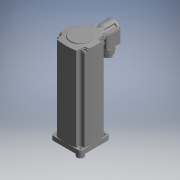
# Autodesk Inventor part: 4808568 EMMT-AS-60-LB---(high_h)
Saved by Autodesk Inventor 2017.3 (Build 213256000, 256)
## iProperties
Part Number: 4808568 EMMT-AS-60-LB---(high_h)
Material: Generic
Catalog Web Link: www.cadenas.de
Description: EMMT-AS (H)-servo motor
Vendor: FESTO
Document SubType Name: Modeling
Designer: partserver
Manufacturer: FESTO
Mass: 654.326 g
Surface Area: 634.047 cm^2
Volume: 654.326 cm^3
Density: 1 g/cm^3
Appearance: PSOLRGB-175-175-175
Category: PARTsolutions
Company: FESTO
Title: 4808568 EMMT-AS-60-LB---(high_h)
Author: Cadenas PARTsolutions
Comments: servo motor
PSOL_IDENT_0: {$CADENAS_DATA\23d-libs\festo\parts\e\emmt\parts\emmt_as.prj},229 {VTYP=3D},{NB=4808568 EMMT-AS-60-L
PSOL_IDENT_1: B---(high_h)},{LINA=4808568 EMMT-AS-60-LB---(high_h)},{NN=EMMT-AS (H)},{DATE=10.08.2021 16:37:16},{G
PSOL_IDENT_2: EOMDATE=08.06.2021 12:24:00},{VERSION=},{LINEID=10},{WBVAR=BAU,WEL,BRE,LODLEVEL},{WBNUMERIC=}  {NB=4
PSOL_IDENT_3: 808568 EMMT-AS-60-LB---(high_h)},{LINA=4808568 EMMT-AS-60-LB---(high_h)},{KT=DUMMY},{TNR=4808568},{T
PSOL_IDENT_4: YP=EMMT-AS},{FLA=60},{BAU=L},{WEL=-},{BRE=B},{LODDEST=mechanical},{LODLEVEL=high},{LODLEVELX='high',
PSOL_IDENT_5: 'High', 'medium', 'Medium','low','Low'},{B1=62},{B2=28},{D1=14},{D2=15},{D3=50},{D4=5},{D5=4.300},{
PSOL_IDENT_6: D6=70},{H1=102},{H3=57},{L=217.300},{L1=187.300},{L2=30},{L3=2.500},{L4=9},{L5=18.400},{L6=44.700},{
PSOL_IDENT_7: L7=14.000},{T1=12.500},{R1=6.000},{WELNB=},{BRENB=B},{BAU1='S','M','L'},{A1=59.000},{R2=90.000},{R3=
PSOL_IDENT_8: 4.000},{R4=0.750},{A2=3.500},{A3=41.274},{R5=1.000},{R6=22.100},{R7=16.900},{R8=15.000},{A4=6.400},{
PSOL_IDENT_9: A5=28.500},{A6=26.500},{A7=4.000},{R9=4.400},{A8=2.400},{R10=2.650},{A9=17.000},{A10=5.500},{R11=2.5
PSOL_IDENT_10: 00},{A11=17.000},{A12=9.000},{Y1=35.000},{X1=52.400},{R12=3.300},{T2=3.400},{T3=1.000},{R13=2.750},{
PSOL_IDENT_11: T4=8.800},{Y2=6.400},{H4=2.400},{H5=31.500},{Y3=31.900},{Y4=8.500},{Y5=13.880},{A13=1.500},{A14=0.35
PSOL_IDENT_12: 0},{A15=1.000},{SC1=1.600}
NB: 4808568 EMMT-AS-60-LB---(high_h)
NN: EMMT-AS (H)
NT: servo motor
NBSYN: $TNR. $TYP.-$FLA.-$BAU.$WELNB.$BRENB.---($LODLEVEL._h)
LINA: 4808568 EMMT-AS-60-LB---(high_h)
CATALOG: Festo
TNR: 4808568
TYP: EMMT-AS
FLA: 60
BAU: L
WEL: -
BRE: B
LODLEVEL: High
B1: 62
B2: 28
D1: 14
D2: 15
D3: 50
D4: 5
D5: 4.3
D6: 70
H1: 102
H3: 57
L2: 30
L3: 2.5
L4: 9
L5: 18.4
L6: 44.7
L7: 14
T1: 12.5
R1: 6
A1: 59
R2: 90
R3: 4
R4: 0.75
A2: 3.5
A3: 41.274
R5: 1
R6: 22.1
R7: 16.9
R8: 15
A4: 6.4
A5: 28.5
A6: 26.5
A7: 4
R9: 4.4
A8: 2.4
R10: 2.65
A9: 17
A10: 5.5
R11: 2.5
A11: 17
A12: 9
Y1: 35
X1: 52.4
R12: 3.3
T2: 3.4
T3: 1
R13: 2.75
T4: 8.8
Y2: 6.4
H4: 2.4
H5: 31.5
Y3: 31.9
Y4: 8.5
Y5: 13.88
A13: 1.5
A14: 0.35
A15: 1
SC1: 1.6
SUPPLIER: FESTO
ARTICLENO: 4808568 EMMT-AS-60-LB---(high_h)
BOMINFO: 4808568 EMMT-AS-60-LB---(high_h)
CREATOR: CADENAS GmbH
Autodesk Inventor part; units mm, degrees
sketch "Sketch_1" plane through (0, 0, 0) normal (0, 0, 1) x (1, 0, 0)
  line L0 (-31, 25) -> (-31, -25)
  arc A0 (-31, -25) -> (-25, -31) centre (-25, -25) ccw
  line L1 (-25, -31) -> (25, -31)
  arc A1 (25, -31) -> (31, -25) centre (25, -25) ccw
  line L2 (31, -25) -> (31, 25)
  arc A2 (31, 25) -> (25, 31) centre (25, 25) ccw
  line L3 (25, 31) -> (-25, 31)
  arc A3 (-25, 31) -> (-31, 25) centre (-25, 25) ccw
  constraints: 8 end point, 8 point on circle, 4 centre point
extrude "Extrusion1" add sketch "Sketch_1" against normal blind 9
sketch "Sketch_2" plane through (0, 0, 0) normal (0.7071068, -0.7071068, 0) x (0, 0, -1)
  line L0 (9, 35) -> (0, 35)
  line L1 (0, 35) -> (0, 37.65)
  line L2 (0, 37.65) -> (0.5, 37.15)
  line L3 (0.5, 37.15) -> (8.5, 37.15)
  line L4 (8.5, 37.15) -> (9, 37.65)
  line L5 (9, 37.65) -> (9, 35)
  line L6 (9, 35) -> (0, 35)
  constraints: 14 end point
revolve "Revolution1" cut sketch "Sketch_2" angle 360 about axis through (24.7487, 24.7487, -9) along (0, 0, -1)
pattern_linear "Rectangular Pattern1" count 2 spacing 49.4975 along (-1, 0, 0) count 2 spacing 49.4975 along (0, -1, 0) of "Revolution1"
sketch "Sketch_4" plane through (0, 0, -9) normal (0, 0, 1) x (1, 0, 0)
  arc A0 (-28.8206, 19.686) -> (-28.8206, -19.686) centre (59, 0) ccw
  arc A1 (-28.8206, -19.686) -> (-28.1932, -20.2647) centre (-28.0888, -19.522) ccw
  line L0 (-28.1932, -20.2647) -> (-23.6462, -20.9037)
  arc A2 (-20.9037, -23.6462) -> (-23.6462, -20.9037) centre (-24.7487, -24.7487) ccw
  line L1 (-20.9037, -23.6462) -> (-20.2647, -28.1932)
  arc A3 (-20.2647, -28.1932) -> (-19.686, -28.8206) centre (-19.522, -28.0888) ccw
  arc A4 (-19.686, -28.8206) -> (19.686, -28.8206) centre (0, 59) ccw
  arc A5 (19.686, -28.8206) -> (20.2647, -28.1932) centre (19.522, -28.0888) ccw
  line L2 (20.2647, -28.1932) -> (20.9037, -23.6462)
  arc A6 (23.6462, -20.9037) -> (20.9037, -23.6462) centre (24.7487, -24.7487) ccw
  line L3 (23.6462, -20.9037) -> (28.1932, -20.2647)
  arc A7 (28.1932, -20.2647) -> (28.8206, -19.686) centre (28.0888, -19.522) ccw
  arc A8 (28.8206, -19.686) -> (28.8206, 19.686) centre (-59, 0) ccw
  arc A9 (28.8206, 19.686) -> (28.1932, 20.2647) centre (28.0888, 19.522) ccw
  line L4 (28.1932, 20.2647) -> (23.6462, 20.9037)
  arc A10 (20.9037, 23.6462) -> (23.6462, 20.9037) centre (24.7487, 24.7487) ccw
  line L5 (20.9037, 23.6462) -> (20.2647, 28.1932)
  arc A11 (20.2647, 28.1932) -> (19.686, 28.8206) centre (19.522, 28.0888) ccw
  arc A12 (19.686, 28.8206) -> (-19.686, 28.8206) centre (0, -59) ccw
  arc A13 (-19.686, 28.8206) -> (-20.2647, 28.1932) centre (-19.522, 28.0888) ccw
  line L6 (-20.2647, 28.1932) -> (-20.9037, 23.6462)
  arc A14 (-23.6462, 20.9037) -> (-20.9037, 23.6462) centre (-24.7487, 24.7487) ccw
  line L7 (-23.6462, 20.9037) -> (-28.1932, 20.2647)
  arc A15 (-28.1932, 20.2647) -> (-28.8206, 19.686) centre (-28.0888, 19.522) ccw
  constraints: 32 point on circle, 16 centre point, 16 end point
extrude "Extrusion2" add sketch "Sketch_4" against normal blind 178.3
sketch "Sketch_5" plane through (0, 0, 0) normal (1, 0, 0) x (0, 1, 0)
  line L0 (0, -187.3) -> (0, -183.8)
  line L1 (42.2, -183.8) -> (37.2, -183.8)
  line L2 (37.2, -183.8) -> (21.5433, -185.2731)
  arc A0 (21.5433, -185.2731) -> (20.637, -186.2687) centre (21.637, -186.2687) ccw
  line L3 (20.637, -186.2687) -> (20.637, -186.8)
  arc A1 (20.137, -187.3) -> (20.637, -186.8) centre (20.137, -186.8) ccw
  line L4 (20.137, -187.3) -> (42.2, -187.3)
  line L5 (42.2, -187.3) -> (42.2, -183.8)
  constraints: 12 end point, 4 point on circle, 2 centre point
revolve "Revolution2" cut sketch "Sketch_5" angle 360 about axis through (0, 0, -187.3) along (0, 0, -1)
sketch "Sketch_9" plane through (0, 0, 0) normal (1, 0, 0) x (0, 1, 0)
  line L0 (0, 0) -> (0, 2.5)
  arc A0 (22.35, 2.5) -> (22.1, 2.25) centre (22.35, 2.25) ccw
  line L1 (22.1, 2.25) -> (22.1, 1)
  line L2 (22.1, 1) -> (16.9, 1)
  line L3 (16.9, 1) -> (16.9, 2.25)
  arc A1 (16.9, 2.25) -> (16.65, 2.5) centre (16.65, 2.25) ccw
  line L4 (16.65, 2.5) -> (15.7, 2.5)
  line L5 (15.7, 2.5) -> (15, 1)
  line L6 (15, 1) -> (15, 0)
  line L7 (15, 0) -> (25, 0)
  line L8 (25, 0) -> (25, 2)
  line L9 (25, 2) -> (24.7, 2.5)
  line L10 (24.7, 2.5) -> (22.35, 2.5)
  constraints: 22 end point, 4 point on circle, 2 centre point
revolve "Revolution3" add sketch "Sketch_9" angle 360 about axis through (0, 0, 0) along (0, 0, -1)
sketch "Sketch_22" plane through (0, 0, 0) normal (1, 0, 0) x (0, 1, 0)
  line L0 (0, -6.4) -> (0, 2.5)
  line L1 (0, 2.5) -> (15, 2.5)
  line L2 (15, 2.5) -> (15, -4.9)
  line L3 (15, -4.9) -> (13.25, -4.9)
  arc A0 (13.25, -4.9) -> (13, -5.15) centre (13.25, -5.15) ccw
  line L4 (13, -5.15) -> (13, -6.4)
  line L5 (13, -6.4) -> (0, -6.4)
  line L6 (0, -6.4) -> (0, 2.5)
  constraints: 14 end point, 2 point on circle, 1 centre point
revolve "Revolution4" cut sketch "Sketch_22" angle 360 about axis through (0, 0, -6.4) along (0, 0, -1)
sketch "Sketch_7" plane through (0, 0, 0) normal (1, 0, 0) x (0, 1, 0)
  line L0 (0, -6.4) -> (0, 11.8066)
  line L1 (0, 11.8066) -> (2.067, 13)
  line L2 (2.067, 13) -> (2.067, 25.567)
  line L3 (2.067, 25.567) -> (2.5, 26)
  line L4 (2.5, 26) -> (2.65, 26)
  line L5 (2.65, 26) -> (2.65, 27.6)
  line L6 (2.65, 27.6) -> (4.05, 29.7979)
  line L7 (4.05, 29.7979) -> (4.4, 30)
  line L8 (4.4, 30) -> (6.6, 30)
  line L9 (6.6, 30) -> (7, 29.6)
  line L10 (7, 29.6) -> (7, 3.5)
  line L11 (7, 3.5) -> (6.8136, 2.8045)
  arc A0 (6.8136, 2.8045) -> (6.8, 2.7009) centre (7.2, 2.7009) ccw
  line L12 (6.8, 2.7009) -> (6.8, 1.9)
  arc A1 (6.8, 1.9) -> (7.2, 1.5) centre (7.2, 1.9) ccw
  line L13 (7.2, 1.5) -> (7.3, 1.5)
  arc A2 (7.5, 1.3) -> (7.3, 1.5) centre (7.3, 1.3) ccw
  line L14 (7.5, 1.3) -> (7.5, -6.4)
  line L15 (7.5, -6.4) -> (0, -6.4)
  line L16 (0, -6.4) -> (0, 11.8066)
  constraints: 34 end point, 6 point on circle, 3 centre point
revolve "Revolution5" add sketch "Sketch_7" angle 360 about axis through (0, 0, -6.4) along (0, 0, -1)
thread "Thread1" size "M5x0.8" class "6H" standard "ISO Metric profile" length 12.5 offset 0.5
sketch "Sketch_10" plane through (0, 0, 0) normal (0, 0, 1) x (1, 0, 0)
  arc A0 (-11.05, 19.1392) -> (-8.45, 14.6358) centre (-9.75, 16.8875) ccw
  arc A1 (8.45, 14.6358) -> (-8.45, 14.6358) centre (0, 0) ccw
  arc A2 (8.45, 14.6358) -> (11.05, 19.1392) centre (9.75, 16.8875) ccw
  arc A3 (11.05, 19.1392) -> (-11.05, 19.1392) centre (0, 0) ccw
  constraints: 8 point on circle, 4 centre point
extrude "Extrusion3" cut sketch "Sketch_10" along normal mid plane 8.8
sketch "Sketch_11" plane through (0, 0, 0) normal (0, 0, 1) x (1, 0, 0)
  arc A0 (-19.1392, 11.05) -> (-19.1392, -11.05) centre (0, 0) ccw
  arc A1 (-19.1392, -11.05) -> (-14.6358, -8.45) centre (-16.8875, -9.75) ccw
  arc A2 (-14.6358, 8.45) -> (-14.6358, -8.45) centre (0, 0) ccw
  arc A3 (-14.6358, 8.45) -> (-19.1392, 11.05) centre (-16.8875, 9.75) ccw
  constraints: 8 point on circle, 4 centre point
extrude "Extrusion4" cut sketch "Sketch_11" along normal mid plane 8.8
sketch "Sketch_12" plane through (0, 0, 0) normal (0, 0, 1) x (1, 0, 0)
  arc A0 (-8.45, -14.6358) -> (-11.05, -19.1392) centre (-9.75, -16.8875) ccw
  arc A1 (-11.05, -19.1392) -> (11.05, -19.1392) centre (0, 0) ccw
  arc A2 (11.05, -19.1392) -> (8.45, -14.6358) centre (9.75, -16.8875) ccw
  arc A3 (-8.45, -14.6358) -> (8.45, -14.6358) centre (0, 0) ccw
  constraints: 8 point on circle, 4 centre point
extrude "Extrusion5" cut sketch "Sketch_12" along normal mid plane 8.8
sketch "Sketch_13" plane through (0, 0, 0) normal (0, 0, 1) x (1, 0, 0)
  arc A0 (14.6358, -8.45) -> (19.1392, -11.05) centre (16.8875, -9.75) ccw
  arc A1 (19.1392, -11.05) -> (19.1392, 11.05) centre (0, 0) ccw
  arc A2 (19.1392, 11.05) -> (14.6358, 8.45) centre (16.8875, 9.75) ccw
  arc A3 (14.6358, -8.45) -> (14.6358, 8.45) centre (0, 0) ccw
  constraints: 8 point on circle, 4 centre point
extrude "Extrusion6" cut sketch "Sketch_13" along normal mid plane 8.8
sketch "Sketch_14" plane through (0, 17.5, 0) normal (0, 1, 0) x (1, 0, 0)
  line L0 (26.2, 0) -> (26.2, 1)
  line L1 (26.2, 1) -> (28.4651, 1)
  arc A0 (28.4651, 1) -> (28.764, 1.2739) centre (28.4651, 1.3) ccw
  line L2 (28.764, 1.2739) -> (28.95, 3.4)
  line L3 (28.95, 3.4) -> (29.5, 3.4)
  line L4 (29.5, 3.4) -> (29.5, 0.5)
  line L5 (29.5, 0.5) -> (30, 0)
  line L6 (30, 0) -> (26.2, 0)
  line L7 (26.2, 0) -> (26.2, 1)
  constraints: 16 end point, 2 point on circle, 1 centre point
revolve "Revolution6" cut sketch "Sketch_14" angle 360 about axis through (26.2, 17.5, 0) along (0, 0, 1)
pattern_linear "Rectangular Pattern2" count 2 spacing 52.4 along (-1, 0, 0) count 2 spacing 35 along (0, -1, 0) of "Revolution6"
sketch "Sketch_16" plane through (0, 0, 0) normal (0, 0, 1) x (1, 0, 0)
  arc A0 (25.0379, 17.1436) -> (25.3103, 16.6718) centre (25.2301, 16.94) ccw
  arc A1 (25.9276, 16.3154) -> (25.3103, 16.6718) centre (25.4508, 16.2023) ccw
  arc A2 (25.9276, 16.3154) -> (26.4724, 16.3154) centre (26.2, 16.38) ccw
  arc A3 (27.0897, 16.6718) -> (26.4724, 16.3154) centre (26.9492, 16.2023) ccw
  arc A4 (27.0897, 16.6718) -> (27.3621, 17.1436) centre (27.1699, 16.94) ccw
  arc A5 (27.3621, 17.8564) -> (27.3621, 17.1436) centre (27.6984, 17.5) ccw
  arc A6 (27.3621, 17.8564) -> (27.0897, 18.3282) centre (27.1699, 18.06) ccw
  arc A7 (26.4724, 18.6846) -> (27.0897, 18.3282) centre (26.9492, 18.7977) ccw
  arc A8 (26.4724, 18.6846) -> (25.9276, 18.6846) centre (26.2, 18.62) ccw
  arc A9 (25.3103, 18.3282) -> (25.9276, 18.6846) centre (25.4508, 18.7977) ccw
  arc A10 (25.3103, 18.3282) -> (25.0379, 17.8564) centre (25.2301, 18.06) ccw
  arc A11 (25.0379, 17.1436) -> (25.0379, 17.8564) centre (24.7016, 17.5) ccw
  constraints: 24 point on circle, 12 centre point
extrude "Extrusion7" cut sketch "Sketch_16" against normal blind 2.25
pattern_linear "Rectangular Pattern3" count 2 spacing 52.4 along (-1, 0, 0) count 2 spacing 35 along (0, -1, 0) of "Extrusion7"
sketch "Sketch_18" plane through (0, 0, -187.3) normal (0, 0, 1) x (1, 0, 0)
  line L0 (-36, -36) -> (36, -36)
  line L1 (36, -36) -> (36, 36)
  line L2 (36, 36) -> (-36, 36)
  line L3 (-36, 36) -> (-36, -36)
  arc A0 (-32.2659, 11.5991) -> (-32.2659, -11.5991) centre (59, 0) ccw
  arc A1 (-32.2659, -11.5991) -> (-31.6262, -12.2472) centre (-31.5219, -11.5045) ccw
  line L4 (-31.6262, -12.2472) -> (-25.0296, -13.1743)
  arc A2 (-21.9443, -16.2596) -> (-25.0296, -13.1743) centre (-26.27, -17.5) ccw
  line L5 (-21.9443, -16.2596) -> (-19.9703, -30.3056)
  arc A3 (-19.9703, -30.3056) -> (-19.3856, -30.9344) centre (-19.2276, -30.2012) ccw
  arc A4 (-19.3856, -30.9344) -> (19.3856, -30.9344) centre (0, 59) ccw
  arc A5 (19.3856, -30.9344) -> (19.9703, -30.3056) centre (19.2276, -30.2012) ccw
  line L6 (19.9703, -30.3056) -> (21.9443, -16.2596)
  arc A6 (25.0296, -13.1743) -> (21.9443, -16.2596) centre (26.27, -17.5) ccw
  line L7 (25.0296, -13.1743) -> (31.6262, -12.2472)
  arc A7 (31.6262, -12.2472) -> (32.2659, -11.5991) centre (31.5219, -11.5045) ccw
  arc A8 (32.2659, -11.5991) -> (32.2659, 11.5991) centre (-59, 0) ccw
  arc A9 (32.2659, 11.5991) -> (31.6262, 12.2472) centre (31.5219, 11.5045) ccw
  line L8 (31.6262, 12.2472) -> (25.0296, 13.1743)
  arc A10 (21.9443, 16.2596) -> (25.0296, 13.1743) centre (26.27, 17.5) ccw
  line L9 (21.9443, 16.2596) -> (19.9703, 30.3056)
  arc A11 (19.9703, 30.3056) -> (19.3856, 30.9344) centre (19.2276, 30.2012) ccw
  arc A12 (19.3856, 30.9344) -> (-19.3856, 30.9344) centre (0, -59) ccw
  arc A13 (-19.3856, 30.9344) -> (-19.9703, 30.3056) centre (-19.2276, 30.2012) ccw
  line L10 (-19.9703, 30.3056) -> (-21.9443, 16.2596)
  arc A14 (-25.0296, 13.1743) -> (-21.9443, 16.2596) centre (-26.27, 17.5) ccw
  line L11 (-25.0296, 13.1743) -> (-31.6262, 12.2472)
  arc A15 (-31.6262, 12.2472) -> (-32.2659, 11.5991) centre (-31.5219, 11.5045) ccw
  constraints: 32 point on circle, 24 end point, 16 centre point
extrude "Extrusion8" cut sketch "Sketch_18" along normal blind 4.5
sketch "Sketch_61" plane through (0, 0, -187.3) normal (0, 0, 1) x (1, 0, 0)
  arc A0 (24.3717, 20.2473) -> (28.5534, 15.1867) centre (26.2, 17.5) ccw
  arc A1 (29.8281, 14.7841) -> (28.5534, 15.1867) centre (29.0883, 14.6609) ccw
  arc A2 (29.8281, 14.7841) -> (28.68, 20.5237) centre (-59, 0) ccw
  line L0 (28.68, 20.5237) -> (24.1815, 21.1559)
  arc A3 (24.3717, 20.2473) -> (24.1815, 21.1559) centre (24.0947, 20.6635) ccw
  constraints: 8 point on circle, 4 centre point, 2 end point
extrude "Extrusion9" cut sketch "Sketch_61" along normal blind 8.8
sketch "Sketch_19" plane through (0, 0, -187.3) normal (0, 0, 1) x (1, 0, 0)
  arc A0 (-28.5534, 15.1867) -> (-29.8281, 14.7841) centre (-29.0883, 14.6609) ccw
  arc A1 (-28.5534, 15.1867) -> (-24.3717, 20.2473) centre (-26.2, 17.5) ccw
  arc A2 (-24.1815, 21.1559) -> (-24.3717, 20.2473) centre (-24.0947, 20.6635) ccw
  line L0 (-24.1815, 21.1559) -> (-28.68, 20.5237)
  arc A3 (-28.68, 20.5237) -> (-29.8281, 14.7841) centre (59, 0) ccw
  constraints: 8 point on circle, 4 centre point, 2 end point
extrude "Extrusion10" cut sketch "Sketch_19" along normal blind 8.8
sketch "Sketch_20" plane through (0, 0, -187.3) normal (0, 0, 1) x (1, 0, 0)
  arc A0 (28.5534, -15.1867) -> (24.3717, -20.2473) centre (26.2, -17.5) ccw
  arc A1 (24.1815, -21.1559) -> (24.3717, -20.2473) centre (24.0947, -20.6635) ccw
  line L0 (24.1815, -21.1559) -> (28.68, -20.5237)
  arc A2 (28.68, -20.5237) -> (29.8281, -14.7841) centre (-59, 0) ccw
  arc A3 (28.5534, -15.1867) -> (29.8281, -14.7841) centre (29.0883, -14.6609) ccw
  constraints: 8 point on circle, 4 centre point, 2 end point
extrude "Extrusion11" cut sketch "Sketch_20" along normal blind 8.8
sketch "Sketch_21" plane through (0, 0, -187.3) normal (0, 0, 1) x (1, 0, 0)
  arc A0 (-29.8281, -14.7841) -> (-28.68, -20.5237) centre (59, 0) ccw
  line L0 (-28.68, -20.5237) -> (-24.1815, -21.1559)
  arc A1 (-24.3717, -20.2473) -> (-24.1815, -21.1559) centre (-24.0947, -20.6635) ccw
  arc A2 (-24.3717, -20.2473) -> (-28.5534, -15.1867) centre (-26.2, -17.5) ccw
  arc A3 (-29.8281, -14.7841) -> (-28.5534, -15.1867) centre (-29.0883, -14.6609) ccw
  constraints: 8 point on circle, 4 centre point, 2 end point
extrude "Extrusion12" cut sketch "Sketch_21" along normal blind 8.8
sketch "Sketch_23" plane through (0, 17.5, 0) normal (0, 1, 0) x (1, 0, 0)
  line L0 (26.2, 178.5) -> (26.2, 180.9)
  line L1 (26.2, 180.9) -> (28.4651, 180.9)
  arc A0 (28.764, 180.6261) -> (28.4651, 180.9) centre (28.4651, 180.6) ccw
  line L2 (28.764, 180.6261) -> (28.95, 178.5)
  line L3 (28.95, 178.5) -> (26.2, 178.5)
  line L4 (26.2, 178.5) -> (26.2, 180.9)
  constraints: 10 end point, 2 point on circle, 1 centre point
revolve "Revolution7" add sketch "Sketch_23" angle 360 about axis through (26.2, 17.5, -178.5) along (0, 0, 1)
pattern_linear "Rectangular Pattern4" count 2 spacing 52.4 along (-1, 0, 0) count 2 spacing 35 along (0, -1, 0) of "Revolution7"
sketch "Sketch_25" plane through (0, 0, -180.9) normal (0, 0, 1) x (1, 0, 0)
  arc A0 (25.0379, 17.1436) -> (25.3103, 16.6718) centre (25.2301, 16.94) ccw
  arc A1 (25.9276, 16.3154) -> (25.3103, 16.6718) centre (25.4508, 16.2023) ccw
  arc A2 (25.9276, 16.3154) -> (26.4724, 16.3154) centre (26.2, 16.38) ccw
  arc A3 (27.0897, 16.6718) -> (26.4724, 16.3154) centre (26.9492, 16.2023) ccw
  arc A4 (27.0897, 16.6718) -> (27.3621, 17.1436) centre (27.1699, 16.94) ccw
  arc A5 (27.3621, 17.8564) -> (27.3621, 17.1436) centre (27.6984, 17.5) ccw
  arc A6 (27.3621, 17.8564) -> (27.0897, 18.3282) centre (27.1699, 18.06) ccw
  arc A7 (26.4724, 18.6846) -> (27.0897, 18.3282) centre (26.9492, 18.7977) ccw
  arc A8 (26.4724, 18.6846) -> (25.9276, 18.6846) centre (26.2, 18.62) ccw
  arc A9 (25.3103, 18.3282) -> (25.9276, 18.6846) centre (25.4508, 18.7977) ccw
  arc A10 (25.3103, 18.3282) -> (25.0379, 17.8564) centre (25.2301, 18.06) ccw
  arc A11 (25.0379, 17.1436) -> (25.0379, 17.8564) centre (24.7016, 17.5) ccw
  constraints: 24 point on circle, 12 centre point
extrude "Extrusion13" cut sketch "Sketch_25" along normal blind 1.3
pattern_linear "Rectangular Pattern5" count 2 spacing 52.4 along (-1, 0, 0) count 2 spacing 35 along (0, -1, 0) of "Extrusion13"
sketch "Sketch_27" plane through (0, 0, 0) normal (0, 1, 0) x (-1, 0, 0)
  arc A0 (13.5, -158.4) -> (10.5, -155.4) centre (10.5, -158.4) ccw
  line L0 (10.5, -155.4) -> (-10.5, -155.4)
  arc A1 (-10.5, -155.4) -> (-13.5, -158.4) centre (-10.5, -158.4) ccw
  line L1 (-13.5, -158.4) -> (-13.5, -179.4)
  arc A2 (-13.5, -179.4) -> (-10.5, -182.4) centre (-10.5, -179.4) ccw
  line L2 (-10.5, -182.4) -> (10.5, -182.4)
  arc A3 (10.5, -182.4) -> (13.5, -179.4) centre (10.5, -179.4) ccw
  line L3 (13.5, -179.4) -> (13.5, -158.4)
  constraints: 8 end point, 8 point on circle, 4 centre point
extrude "Extrusion14" add sketch "Sketch_27" along normal blind 31.5
sketch "Sketch_28" plane through (0, 31.5, 0) normal (0, 1, 0) x (1, 0, 0)
  arc A0 (-13, 158.92) -> (-10, 155.92) centre (-10, 158.92) ccw
  line L0 (-10, 155.92) -> (10, 155.92)
  arc A1 (10, 155.92) -> (13, 158.92) centre (10, 158.92) ccw
  line L1 (13, 158.92) -> (13, 178.92)
  arc A2 (13, 178.92) -> (10, 181.92) centre (10, 178.92) ccw
  line L2 (10, 181.92) -> (-10, 181.92)
  arc A3 (-10, 181.92) -> (-13, 178.92) centre (-10, 178.92) ccw
  line L3 (-13, 178.92) -> (-13, 158.92)
  constraints: 8 end point, 8 point on circle, 4 centre point
extrude "Extrusion15" add sketch "Sketch_28" along normal blind 4.65
sketch "Sketch_29" plane through (0, 0, 0) normal (1, 0, 0) x (0, 1, 0)
  line L0 (36.15, -168.9) -> (71, -168.9)
  line L1 (71, -168.9) -> (71, -179.9)
  arc A0 (68, -182.9) -> (71, -179.9) centre (68, -179.9) ccw
  line L2 (68, -182.9) -> (47.65, -182.9)
  arc A1 (41.65, -180.9) -> (47.65, -182.9) centre (48.9628, -168.9617) ccw
  line L3 (41.65, -180.9) -> (41.65, -180.8)
  line L4 (41.65, -180.8) -> (38.7, -180.8)
  arc A2 (38.7, -180.8) -> (38.4, -181.1) centre (38.7, -181.1) ccw
  arc A3 (36.15, -181.9) -> (38.4, -181.1) centre (35.9961, -177.903) ccw
  line L5 (36.15, -181.9) -> (36.15, -168.9)
  line L6 (36.15, -168.9) -> (71, -168.9)
  constraints: 14 end point, 8 point on circle, 4 centre point
revolve "Revolution8" add sketch "Sketch_29" angle 360 about axis through (0, 36.15, -168.9) along (0, -1, 0)
sketch "Sketch_34" plane through (0, 0, -168.9) normal (0, 0, 1) x (1, 0, 0)
  line L0 (-14, 68) -> (-14, 47.65)
  arc A0 (-14, 47.65) -> (-12, 41.65) centre (-0.0617, 48.9628) ccw
  line L1 (-12, 41.65) -> (12, 41.65)
  arc A1 (12, 41.65) -> (14, 47.65) centre (0.0617, 48.9628) ccw
  line L2 (14, 47.65) -> (14, 68)
  arc A2 (14, 68) -> (11, 71) centre (11, 68) ccw
  line L3 (11, 71) -> (-11, 71)
  arc A3 (-11, 71) -> (-14, 68) centre (-11, 68) ccw
  constraints: 8 end point, 8 point on circle, 4 centre point
extrude "Extrusion16" add sketch "Sketch_34" along normal blind 23.8
sketch "Sketch_30" plane through (0, 36.15, 0) normal (0, 1, 0) x (1, 0, 0)
  circle A0 centre (9.9, 178.8) radius 3.3
  constraints: 1 centre point
extrude "Extrusion17" cut sketch "Sketch_30" along normal blind 28.2
sketch "Sketch_31" plane through (0, 36.15, 0) normal (0, 1, 0) x (1, 0, 0)
  circle A0 centre (-9.9, 178.8) radius 3.3
  constraints: 1 centre point
extrude "Extrusion18" cut sketch "Sketch_31" along normal blind 28.2
sketch "Sketch_32" plane through (0, 36.15, 0) normal (0, 1, 0) x (1, 0, 0)
  circle A0 centre (9.9, 159) radius 3.3
  constraints: 1 centre point
extrude "Extrusion19" cut sketch "Sketch_32" along normal blind 5.5
sketch "Sketch_33" plane through (0, 36.15, 0) normal (0, 1, 0) x (1, 0, 0)
  circle A0 centre (-9.9, 159) radius 3.3
  constraints: 1 centre point
extrude "Extrusion20" cut sketch "Sketch_33" along normal blind 5.5
sketch "Sketch_35" plane through (9.9, 0, 0) normal (1, 0, 0) x (0, 0, -1)
  line L0 (159.02, 36.15) -> (159.02, 38.55)
  line L1 (159.02, 38.55) -> (160.52, 38.55)
  arc A0 (161.9875, 37.9804) -> (160.52, 38.55) centre (160.52, 36.375) ccw
  arc A1 (162.02, 37.9065) -> (161.9875, 37.9804) centre (161.92, 37.9065) ccw
  line L2 (162.02, 37.9065) -> (162.02, 36.15)
  line L3 (162.02, 36.15) -> (159.02, 36.15)
  line L4 (159.02, 36.15) -> (159.02, 38.55)
  constraints: 10 end point, 4 point on circle, 2 centre point
revolve "Revolution9" add sketch "Sketch_35" angle 360 about axis through (9.9, 36.15, -159.02) along (0, -1, 0)
pattern_linear "Rectangular Pattern6" count 2 spacing 19.8 along (0, 0, -1) count 2 spacing 19.8 along (-1, 0, 0) of "Revolution9"
sketch "Sketch_37" plane through (0, 38.55, 0) normal (0, 1, 0) x (1, 0, 0)
  line L0 (7.51, 159.52) -> (7.51, 158.52)
  line L1 (7.51, 158.52) -> (9.0242, 158.52)
  arc A0 (9.0718, 158.1303) -> (9.0242, 158.52) centre (8.6023, 158.2708) ccw
  arc A1 (9.0718, 158.1303) -> (9.5436, 157.8579) centre (9.34, 158.0501) ccw
  arc A2 (10.2564, 157.8579) -> (9.5436, 157.8579) centre (9.9, 157.5216) ccw
  arc A3 (10.2564, 157.8579) -> (10.7282, 158.1303) centre (10.46, 158.0501) ccw
  arc A4 (10.7758, 158.52) -> (10.7282, 158.1303) centre (11.1977, 158.2708) ccw
  line L2 (10.7758, 158.52) -> (12.29, 158.52)
  line L3 (12.29, 158.52) -> (12.29, 159.52)
  line L4 (12.29, 159.52) -> (10.7758, 159.52)
  arc A5 (10.7282, 159.9097) -> (10.7758, 159.52) centre (11.1977, 159.7692) ccw
  arc A6 (10.7282, 159.9097) -> (10.2564, 160.1821) centre (10.46, 159.9899) ccw
  arc A7 (9.5436, 160.1821) -> (10.2564, 160.1821) centre (9.9, 160.5184) ccw
  arc A8 (9.5436, 160.1821) -> (9.0718, 159.9097) centre (9.34, 159.9899) ccw
  arc A9 (9.0242, 159.52) -> (9.0718, 159.9097) centre (8.6023, 159.7692) ccw
  line L5 (9.0242, 159.52) -> (7.51, 159.52)
  constraints: 20 point on circle, 12 end point, 10 centre point
extrude "Extrusion21" cut sketch "Sketch_37" against normal blind 1.3
pattern_linear "Rectangular Pattern7" count 2 spacing 19.8 along (0, 0, -1) count 2 spacing 19.8 along (-1, 0, 0) of "Extrusion21"
sketch "Sketch_39" plane through (0, 68, 0) normal (0, 1, 0) x (1, 0, 0)
  arc A0 (8.7579, 176.2928) -> (11.3421, 170.5472) centre (10.05, 173.42) ccw
  line L0 (11.3421, 170.5472) -> (13.7328, 171.6224)
  arc A1 (13.7328, 171.6224) -> (11.1486, 177.368) centre (0, 168.9) ccw
  line L1 (11.1486, 177.368) -> (8.7579, 176.2928)
  constraints: 4 end point, 4 point on circle, 2 centre point
extrude "Extrusion22" cut sketch "Sketch_39" along normal blind 3
sketch "Sketch_40" plane through (0, 68, 0) normal (0, 1, 0) x (1, 0, 0)
  line L0 (-13.7328, 171.6224) -> (-11.3421, 170.5472)
  arc A0 (-11.3421, 170.5472) -> (-8.7579, 176.2928) centre (-10.05, 173.42) ccw
  line L1 (-8.7579, 176.2928) -> (-11.1486, 177.368)
  arc A1 (-11.1486, 177.368) -> (-13.7328, 171.6224) centre (0, 168.9) ccw
  constraints: 4 end point, 4 point on circle, 2 centre point
extrude "Extrusion23" cut sketch "Sketch_40" along normal blind 3
sketch "Sketch_41" plane through (10.05, 0, 0) normal (1, 0, 0) x (0, 0, -1)
  line L0 (173.42, 68) -> (173.42, 70.25)
  line L1 (173.42, 70.25) -> (174.6088, 70.25)
  arc A0 (176.42, 69.6) -> (174.6088, 70.25) centre (173.5139, 64.3507) ccw
  line L2 (176.42, 69.6) -> (176.42, 68)
  line L3 (176.42, 68) -> (173.42, 68)
  line L4 (173.42, 68) -> (173.42, 70.25)
  constraints: 10 end point, 2 point on circle, 1 centre point
revolve "Revolution10" add sketch "Sketch_41" angle 360 about axis through (10.05, 68, -173.42) along (0, -1, 0)
pattern_linear "Rectangular Pattern8" count 2 spacing 20.1 along (-1, 0, 0) of "Revolution10"
sketch "Sketch_43" plane through (0, 70.35, 0) normal (0, 1, 0) x (1, 0, 0)
  arc A0 (8.6804, 173) -> (9.0014, 172.4438) centre (8.9068, 172.76) ccw
  arc A1 (9.7289, 172.0238) -> (9.0014, 172.4438) centre (9.167, 171.8906) ccw
  arc A2 (9.7289, 172.0238) -> (10.3711, 172.0238) centre (10.05, 172.1) ccw
  arc A3 (11.0986, 172.4438) -> (10.3711, 172.0238) centre (10.933, 171.8906) ccw
  arc A4 (11.0986, 172.4438) -> (11.4196, 173) centre (11.1932, 172.76) ccw
  arc A5 (11.4196, 173.84) -> (11.4196, 173) centre (11.816, 173.42) ccw
  arc A6 (11.4196, 173.84) -> (11.0986, 174.3962) centre (11.1932, 174.08) ccw
  arc A7 (10.3711, 174.8162) -> (11.0986, 174.3962) centre (10.933, 174.9494) ccw
  arc A8 (10.3711, 174.8162) -> (9.7289, 174.8162) centre (10.05, 174.74) ccw
  arc A9 (9.0014, 174.3962) -> (9.7289, 174.8162) centre (9.167, 174.9494) ccw
  arc A10 (9.0014, 174.3962) -> (8.6804, 173.84) centre (8.9068, 174.08) ccw
  arc A11 (8.6804, 173) -> (8.6804, 173.84) centre (8.284, 173.42) ccw
  constraints: 24 point on circle, 12 centre point
extrude "Extrusion24" cut sketch "Sketch_43" against normal blind 1.5
pattern_linear "Rectangular Pattern9" count 2 spacing 20.1 along (-1, 0, 0) of "Extrusion24"
sketch "Sketch_45" plane through (0, 0, 0) normal (1, 0, 0) x (0, 1, 0)
  line L0 (57, -145.1) -> (57, -140.34)
  line L1 (57, -140.3) -> (66.225, -140.3)
  line L2 (66.225, -140.3) -> (66.225, -129.2)
  line L3 (66.225, -129.2) -> (66.3982, -128.9)
  line L4 (66.3982, -128.9) -> (67.4863, -128.9)
  line L5 (67.4863, -128.9) -> (67.775, -129.4)
  line L6 (67.775, -129.4) -> (67.775, -134.18)
  line L7 (67.775, -134.18) -> (67.8865, -134.18)
  line L8 (67.8865, -134.18) -> (68.5, -134.7935)
  line L9 (68.5, -134.7935) -> (68.5, -139.7265)
  line L10 (68.5, -139.7265) -> (67.8865, -140.34)
  line L11 (67.8865, -140.34) -> (67.8425, -140.34)
  line L12 (67.8425, -140.34) -> (67.8425, -141.83)
  line L13 (67.8425, -141.83) -> (68.45, -142.05)
  line L14 (68.45, -142.05) -> (68.45, -142.65)
  arc A0 (68.3, -142.8) -> (68.45, -142.65) centre (68.3, -142.65) ccw
  line L15 (68.3, -142.8) -> (67.975, -142.8)
  line L16 (67.975, -142.8) -> (67.975, -143.15)
  arc A1 (67.975, -144.05) -> (67.975, -143.15) centre (68.575, -143.6) ccw
  line L17 (67.975, -144.05) -> (67.975, -144.4)
  line L18 (67.975, -144.4) -> (68.3, -144.4)
  arc A2 (68.45, -144.55) -> (68.3, -144.4) centre (68.3, -144.55) ccw
  line L19 (68.45, -144.55) -> (68.45, -144.95)
  arc A3 (68.45, -144.95) -> (68.6, -145.1) centre (68.6, -144.95) ccw
  line L20 (68.6, -145.1) -> (57, -145.1)
  line L21 (57, -145.1) -> (57, -140.3)
  constraints: 44 end point, 8 point on circle, 4 centre point
revolve "Revolution11" add sketch "Sketch_45" angle 360 about axis through (0, 57, -145.1) along (0, 0, -1)
sketch "Sketch_46" plane through (0, 0, -140.3) normal (0, 0, 1) x (1, 0, 0)
  line L0 (-15, 42) -> (15, 42)
  line L1 (15, 42) -> (15, 72)
  line L2 (15, 72) -> (-15, 72)
  line L3 (-15, 72) -> (-15, 42)
  line L4 (-10.7, 45) -> (10.7, 45)
  line L5 (10.7, 45) -> (10.7, 69)
  line L6 (10.7, 69) -> (-10.7, 69)
  line L7 (-10.7, 69) -> (-10.7, 45)
  constraints: 16 end point
extrude "Extrusion25" cut sketch "Sketch_46" along normal blind 6.2
sketch "Sketch_47" plane through (0, 0, -140.3) normal (0, 0, 1) x (1, 0, 0)
  arc A0 (-9.6245, 57.0957) -> (9.6245, 57.0957) centre (0, 57) ccw
  arc A1 (9.6245, 57.0957) -> (9.254, 57.5737) centre (9.1245, 57.0907) ccw
  line L0 (9.254, 57.5737) -> (7.2319, 58.1155)
  arc A2 (7.2319, 58.1155) -> (6.4684, 58.216) centre (6.4684, 55.266) ccw
  line L1 (6.4684, 58.216) -> (5.2718, 58.216)
  arc A3 (5.2718, 58.216) -> (3.3924, 56.9) centre (5.2718, 56.216) ccw
  line L2 (3.3924, 56.9) -> (2.8039, 55.2832)
  arc A4 (0, 53.25) -> (2.8039, 55.2832) centre (0, 56.2) ccw
  arc A5 (-2.8039, 55.2832) -> (0, 53.25) centre (0, 56.2) ccw
  line L3 (-2.8039, 55.2832) -> (-3.3924, 56.9)
  arc A6 (-3.3924, 56.9) -> (-5.2718, 58.216) centre (-5.2718, 56.216) ccw
  line L4 (-5.2718, 58.216) -> (-6.4684, 58.216)
  arc A7 (-6.4684, 58.216) -> (-7.2319, 58.1155) centre (-6.4684, 55.266) ccw
  line L5 (-7.2319, 58.1155) -> (-9.254, 57.5737)
  arc A8 (-9.254, 57.5737) -> (-9.6245, 57.0957) centre (-9.1245, 57.0907) ccw
  constraints: 18 point on circle, 12 end point, 9 centre point
extrude "Extrusion26" add sketch "Sketch_47" along normal blind 16.1
sketch "Sketch_48" plane through (0, 0, -140.3) normal (0, 0, 1) x (1, 0, 0)
  circle A0 centre (6.4716, 55.2655) radius 2.55
  constraints: 1 centre point
extrude "Extrusion27" cut sketch "Sketch_48" along normal blind 16.1
sketch "Pattern_10_Sketch_48_0" plane through (0, 0, -140.3) normal (0, 0, 1) x (1, 0, 0)
  circle A0 centre (-6.4716, 55.2655) radius 2.55
  constraints: 1 centre point
extrude "Extrusion28" cut sketch "Pattern_10_Sketch_48_0" along normal blind 16.1
sketch "Pattern_10_Sketch_48_1" plane through (0, 0, -140.3) normal (0, 0, 1) x (1, 0, 0)
  circle A0 centre (-2.8306, 50.9273) radius 2.55
  constraints: 1 centre point
extrude "Extrusion29" cut sketch "Pattern_10_Sketch_48_1" along normal blind 16.1
sketch "Pattern_10_Sketch_48_2" plane through (0, 0, -140.3) normal (0, 0, 1) x (1, 0, 0)
  circle A0 centre (2.8306, 50.9273) radius 2.55
  constraints: 1 centre point
extrude "Extrusion30" cut sketch "Pattern_10_Sketch_48_2" along normal blind 16.1
sketch "Sketch_50" plane through (0, 0, -140.3) normal (0, 0, 1) x (1, 0, 0)
  circle A0 centre (6.4716, 55.2655) radius 0.995
  constraints: 1 centre point
extrude "Extrusion31" add sketch "Sketch_50" along normal blind 10.3
sketch "Pattern_11_SKETCH_1" plane through (0, 0, -140.3) normal (0, 0, 1) x (1, 0, 0)
  circle A0 centre (-6.4716, 55.2655) radius 0.995
  constraints: 1 centre point
sketch "Pattern_11_SKETCH_2" plane through (0, 0, -140.3) normal (0, 0, 1) x (1, 0, 0)
  circle A0 centre (-2.8306, 50.9273) radius 0.995
  constraints: 1 centre point
sketch "Pattern_11_SKETCH_3" plane through (0, 0, -140.3) normal (0, 0, 1) x (1, 0, 0)
  circle A0 centre (2.8306, 50.9273) radius 0.995
  constraints: 1 centre point
extrude "Extrusion32" add sketch "Pattern_11_SKETCH_1" along normal blind 10.3
extrude "Extrusion33" add sketch "Pattern_11_SKETCH_2" along normal blind 10.3
extrude "Extrusion34" add sketch "Pattern_11_SKETCH_3" along normal blind 10.3
sketch "Sketch_52" plane through (0, 0, 0) normal (1, 0, 0) x (0, 1, 0)
  line L0 (56.2, -140.3) -> (56.2, -129)
  line L1 (56.2, -129) -> (56.695, -129)
  arc A0 (57.195, -129.5) -> (56.695, -129) centre (56.695, -129.5) ccw
  line L2 (57.195, -129.5) -> (57.195, -140.3)
  line L3 (57.195, -140.3) -> (56.2, -140.3)
  line L4 (56.2, -140.3) -> (56.2, -129)
  constraints: 10 end point, 2 point on circle, 1 centre point
revolve "Revolution12" add sketch "Sketch_52" angle 360 about axis through (0, 56.2, -140.3) along (0, 0, -1)
sketch "Sketch_53" plane through (0, 0, -140.3) normal (0, 0, 1) x (1, 0, 0)
  line L0 (-9.7626, 59.166) -> (-5.01, 59.166)
  arc A0 (-2.5771, 57.8881) -> (-5.01, 59.166) centre (-5.0074, 56.216) ccw
  arc A1 (-2.6742, 57.4583) -> (-2.5771, 57.8881) centre (-2.8242, 57.7181) ccw
  line L1 (-2.6742, 57.4583) -> (-3.741, 56.8423)
  line L2 (-3.741, 56.8423) -> (-2.7421, 55.1121)
  arc A2 (-2.7421, 55.1121) -> (2.7421, 55.1121) centre (0, 56.2) ccw
  line L3 (2.7421, 55.1121) -> (3.741, 56.8423)
  line L4 (3.741, 56.8423) -> (2.6742, 57.4583)
  arc A3 (2.5771, 57.8881) -> (2.6742, 57.4583) centre (2.8242, 57.7181) ccw
  arc A4 (5.01, 59.166) -> (2.5771, 57.8881) centre (5.0074, 56.216) ccw
  line L5 (5.01, 59.166) -> (9.7626, 59.166)
  arc A5 (9.7626, 59.166) -> (-9.7626, 59.166) centre (0, 57) ccw
  constraints: 12 end point, 12 point on circle, 6 centre point
extrude "Extrusion35" add sketch "Sketch_53" along normal blind 3.1
sketch "Sketch_54" plane through (0, 0, -140.3) normal (0, 0, 1) x (1, 0, 0)
  line L0 (-9.7626, 59.166) -> (-5.3804, 59.166)
  arc A0 (-3.5028, 61.6228) -> (-5.3804, 59.166) centre (0, 57) ccw
  arc A1 (3.5028, 61.6228) -> (-3.5028, 61.6228) centre (0, 62.2) ccw
  arc A2 (5.3804, 59.166) -> (3.5028, 61.6228) centre (0, 57) ccw
  line L1 (5.3804, 59.166) -> (9.7626, 59.166)
  arc A3 (9.7626, 59.166) -> (-9.7626, 59.166) centre (0, 57) ccw
  constraints: 8 point on circle, 4 centre point, 4 end point
extrude "Extrusion36" add sketch "Sketch_54" along normal blind 5.1
sketch "Sketch_55" plane through (0, 0, 0) normal (1, 0, 0) x (0, 1, 0)
  line L0 (62.2, -140.3) -> (62.2, -134.675)
  line L1 (62.2, -134.675) -> (64.7, -134.675)
  arc A0 (64.8, -134.775) -> (64.7, -134.675) centre (64.7, -134.775) ccw
  line L2 (64.8, -134.775) -> (64.8, -140.3)
  line L3 (64.8, -140.3) -> (62.2, -140.3)
  line L4 (62.2, -140.3) -> (62.2, -134.675)
  constraints: 10 end point, 2 point on circle, 1 centre point
revolve "Revolution13" add sketch "Sketch_55" angle 360 about axis through (0, 62.2, -140.3) along (0, 0, -1)
sketch "Sketch_56" plane through (1.7, 0, 0) normal (1, 0, 0) x (0, 0, -1)
  line L0 (140.3, 62.2) -> (130.775, 62.2)
  arc A0 (131.09, 62.515) -> (130.775, 62.2) centre (131.09, 62.2) ccw
  line L1 (131.09, 62.515) -> (140.3, 62.515)
  line L2 (140.3, 62.515) -> (140.3, 62.2)
  line L3 (140.3, 62.2) -> (130.775, 62.2)
  constraints: 8 end point, 2 point on circle, 1 centre point
revolve "Revolution14" add sketch "Sketch_56" angle 360 about axis through (1.7, 62.2, -140.3) along (0, 0, -1)
sketch "Pattern_12_SKETCH_1" plane through (0.85, 1.472, 0) normal (1, 0, 0) x (0, 0, -1)
  line L0 (140.3, 62.2) -> (130.775, 62.2)
  arc A0 (131.09, 62.515) -> (130.775, 62.2) centre (131.09, 62.2) ccw
  line L1 (131.09, 62.515) -> (140.3, 62.515)
  line L2 (140.3, 62.515) -> (140.3, 62.2)
  line L3 (140.3, 62.2) -> (130.775, 62.2)
  constraints: 8 end point, 2 point on circle, 1 centre point
sketch "Pattern_12_SKETCH_2" plane through (-0.85, 1.472, 0) normal (1, 0, 0) x (0, 0, -1)
  line L0 (140.3, 62.2) -> (130.775, 62.2)
  arc A0 (131.09, 62.515) -> (130.775, 62.2) centre (131.09, 62.2) ccw
  line L1 (131.09, 62.515) -> (140.3, 62.515)
  line L2 (140.3, 62.515) -> (140.3, 62.2)
  line L3 (140.3, 62.2) -> (130.775, 62.2)
  constraints: 8 end point, 2 point on circle, 1 centre point
sketch "Pattern_12_SKETCH_3" plane through (0.85, 1.472, 0) normal (1, 0, 0) x (0, 0, -1)
  line L0 (140.3, 59.25) -> (130.775, 59.25)
  arc A0 (131.09, 59.565) -> (130.775, 59.25) centre (131.09, 59.25) ccw
  line L1 (131.09, 59.565) -> (140.3, 59.565)
  line L2 (140.3, 59.565) -> (140.3, 59.25)
  line L3 (140.3, 59.25) -> (130.775, 59.25)
  constraints: 8 end point, 2 point on circle, 1 centre point
sketch "Pattern_12_SKETCH_4" plane through (-0.85, 1.472, 0) normal (1, 0, 0) x (0, 0, -1)
  line L0 (140.3, 59.25) -> (130.775, 59.25)
  arc A0 (131.09, 59.565) -> (130.775, 59.25) centre (131.09, 59.25) ccw
  line L1 (131.09, 59.565) -> (140.3, 59.565)
  line L2 (140.3, 59.565) -> (140.3, 59.25)
  line L3 (140.3, 59.25) -> (130.775, 59.25)
  constraints: 8 end point, 2 point on circle, 1 centre point
sketch "Pattern_12_SKETCH_5" plane through (-1.7, 0, 0) normal (1, 0, 0) x (0, 0, -1)
  line L0 (140.3, 62.2) -> (130.775, 62.2)
  arc A0 (131.09, 62.515) -> (130.775, 62.2) centre (131.09, 62.2) ccw
  line L1 (131.09, 62.515) -> (140.3, 62.515)
  line L2 (140.3, 62.515) -> (140.3, 62.2)
  line L3 (140.3, 62.2) -> (130.775, 62.2)
  constraints: 8 end point, 2 point on circle, 1 centre point
revolve "Revolution15" add sketch "Pattern_12_SKETCH_1" angle 360 about axis through (0.85, 63.672, -140.3) along (0, 0, -1)
revolve "Revolution16" add sketch "Pattern_12_SKETCH_2" angle 360 about axis through (-0.85, 63.672, -140.3) along (0, 0, -1)
revolve "Revolution17" add sketch "Pattern_12_SKETCH_3" angle 360 about axis through (0.85, 60.722, -140.3) along (0, 0, -1)
revolve "Revolution18" add sketch "Pattern_12_SKETCH_4" angle 360 about axis through (-0.85, 60.722, -140.3) along (0, 0, -1)
revolve "Revolution19" add sketch "Pattern_12_SKETCH_5" angle 360 about axis through (-1.7, 62.2, -140.3) along (0, 0, -1)
sketch "Sketch_58" plane through (6.741, 0, 0) normal (1, 0, 0) x (0, 0, -1)
  line L0 (140.3, 60.287) -> (129.25, 60.287)
  line L1 (129.25, 60.287) -> (129.25, 60.542)
  arc A0 (129.8999, 60.782) -> (129.25, 60.542) centre (129.8999, 59.782) ccw
  line L2 (129.8999, 60.782) -> (140.3, 60.782)
  line L3 (140.3, 60.782) -> (140.3, 60.287)
  line L4 (140.3, 60.287) -> (129.25, 60.287)
  constraints: 10 end point, 2 point on circle, 1 centre point
revolve "Revolution20" add sketch "Sketch_58" angle 360 about axis through (6.741, 60.287, -140.3) along (0, 0, -1)
sketch "Pattern_13_SKETCH_1" plane through (5.0185, 2.286, 0) normal (1, 0, 0) x (0, 0, -1)
  line L0 (140.3, 60.287) -> (129.25, 60.287)
  line L1 (129.25, 60.287) -> (129.25, 60.542)
  arc A0 (129.8999, 60.782) -> (129.25, 60.542) centre (129.8999, 59.782) ccw
  line L2 (129.8999, 60.782) -> (140.3, 60.782)
  line L3 (140.3, 60.782) -> (140.3, 60.287)
  line L4 (140.3, 60.287) -> (129.25, 60.287)
  constraints: 10 end point, 2 point on circle, 1 centre point
sketch "Pattern_13_SKETCH_2" plane through (-5.0185, 2.286, 0) normal (1, 0, 0) x (0, 0, -1)
  line L0 (140.3, 60.287) -> (129.25, 60.287)
  line L1 (129.25, 60.287) -> (129.25, 60.542)
  arc A0 (129.8999, 60.782) -> (129.25, 60.542) centre (129.8999, 59.782) ccw
  line L2 (129.8999, 60.782) -> (140.3, 60.782)
  line L3 (140.3, 60.782) -> (140.3, 60.287)
  line L4 (140.3, 60.287) -> (129.25, 60.287)
  constraints: 10 end point, 2 point on circle, 1 centre point
sketch "Pattern_13_SKETCH_3" plane through (-6.741, 0, 0) normal (1, 0, 0) x (0, 0, -1)
  line L0 (140.3, 60.287) -> (129.25, 60.287)
  line L1 (129.25, 60.287) -> (129.25, 60.542)
  arc A0 (129.8999, 60.782) -> (129.25, 60.542) centre (129.8999, 59.782) ccw
  line L2 (129.8999, 60.782) -> (140.3, 60.782)
  line L3 (140.3, 60.782) -> (140.3, 60.287)
  line L4 (140.3, 60.287) -> (129.25, 60.287)
  constraints: 10 end point, 2 point on circle, 1 centre point
revolve "Revolution21" add sketch "Pattern_13_SKETCH_1" angle 360 about axis through (5.0185, 62.573, -140.3) along (0, 0, -1)
revolve "Revolution22" add sketch "Pattern_13_SKETCH_2" angle 360 about axis through (-5.0185, 62.573, -140.3) along (0, 0, -1)
revolve "Revolution23" add sketch "Pattern_13_SKETCH_3" angle 360 about axis through (-6.741, 60.287, -140.3) along (0, 0, -1)
ref_plane "ANBAU_XY" through (0, 0, 0) normal (0, 0, -1) x (1, 0, 0)
ref_plane "ANBAU_YZ" through (0, 0, 0) normal (1, 0, 0) x (0, -1, 0)
ref_plane "ANBAU_ZX" through (0, 0, 0) normal (0, -1, 0) x (0, 0, -1)
ref_plane "IP1_XY" through (0, 0, -4.9) normal (0, 0, -1) x (1, 0, 0)
ref_plane "IP1_YZ" through (0, 0, -4.9) normal (1, 0, 0) x (0, -1, 0)
ref_plane "IP1_ZX" through (0, 0, -4.9) normal (0, -1, 0) x (0, 0, -1)
ref_plane "LEI_XY" through (0, 57, -145.1) normal (0, 0, 1) x (1, 0, 0)
ref_plane "LEI_YZ" through (0, 57, -145.1) normal (1, 0, 0) x (0, 1, 0)
ref_plane "LEI_ZX" through (0, 57, -145.1) normal (0, 1, 0) x (0, 0, 1)
ref_plane "SCREWS_1_XY" through (24.7487, 24.7487, -9) normal (0, 0, 1) x (1, 0, 0)
ref_plane "SCREWS_1_YZ" through (24.7487, 24.7487, -9) normal (1, 0, 0) x (0, 1, 0)
ref_plane "SCREWS_1_ZX" through (24.7487, 24.7487, -9) normal (0, 1, 0) x (0, 0, 1)
ref_plane "SCREWS_2_XY" through (-24.7487, 24.7487, -9) normal (0, 0, 1) x (1, 0, 0)
ref_plane "SCREWS_2_YZ" through (-24.7487, 24.7487, -9) normal (1, 0, 0) x (0, 1, 0)
ref_plane "SCREWS_2_ZX" through (-24.7487, 24.7487, -9) normal (0, 1, 0) x (0, 0, 1)
ref_plane "SCREWS_3_XY" through (-24.7487, -24.7487, -9) normal (0, 0, 1) x (1, 0, 0)
ref_plane "SCREWS_3_YZ" through (-24.7487, -24.7487, -9) normal (1, 0, 0) x (0, 1, 0)
ref_plane "SCREWS_3_ZX" through (-24.7487, -24.7487, -9) normal (0, 1, 0) x (0, 0, 1)
ref_plane "SCREWS_4_XY" through (24.7487, -24.7487, -9) normal (0, 0, 1) x (1, 0, 0)
ref_plane "SCREWS_4_YZ" through (24.7487, -24.7487, -9) normal (1, 0, 0) x (0, 1, 0)
ref_plane "SCREWS_4_ZX" through (24.7487, -24.7487, -9) normal (0, 1, 0) x (0, 0, 1)
body "Solid1"
